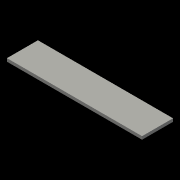
# Autodesk Inventor part: MFLMLMRMFR
Saved by Autodesk Inventor 2016 (Build 200138000, 138)
## iProperties
Created: 2017-01-21
Part Number: MFLMLMRMFR
Material: Generic
Document SubType Name: Modeling
Designer: Alexis Renderos
Density: 1 g/cm^3
Appearance: Ivory Flat
Author: Alexis Renderos
Autodesk Inventor part; units mm, degrees
ref_plane "YZ Plane" through (0, 0, 0) normal (1, 0, 0) x (0, 1, 0)
ref_plane "XZ Plane" through (0, 0, 0) normal (0, 1, 0) x (-1, 0, 0)
ref_plane "XY Plane" through (0, 0, 0) normal (0, 0, 1) x (1, 0, 0)
sketch "Sketch1" plane through (0, 0, 0) normal (0, 1, 0) x (-1, 0, 0)
  line L0 (0, -44.45) -> (0, 44.45) projected
  line L1 (-193.802, 0) -> (193.802, 0) projected
  line L2 (-138.43, 31.75) -> (138.43, 31.75)
  line L3 (138.43, 31.75) -> (138.43, -31.75)
  line L4 (138.43, -31.75) -> (-138.43, -31.75)
  line L5 (-138.43, -31.75) -> (-138.43, 31.75)
  line L6 (-138.43, 31.75) -> (138.43, -31.75) construction
  line L7 (138.43, 31.75) -> (-138.43, -31.75) construction
  point P0 (0, 0)
  dimension "d0" = 276.86
  dimension "d1" = 63.5
  constraints: 12 end point, 2 midpoint, 2 parallel, 1 horizontal, 1 perpendicular
  measures "d0" distance of L3.end L4.end
  measures "d1" distance of L2.end L3.end
extrude "Extrusion1" add sketch "Sketch1" along normal mid plane 6.35
body "Solid1"
